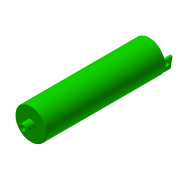
# Autodesk Inventor part: PC3.5-P1
Saved by Autodesk Inventor 2015 (Build 190159000, 159)
## iProperties
Created: 2015-01-13
Part Number: PC3.5-P1
Material: Generic
Document SubType Name: Modeling
Designer: Collin_2
Density: 1 g/cm^3
Appearance: Default
Author: Collin_2
Autodesk Inventor part; units mm, degrees
ref_plane "YZ Plane" through (0, 0, 0) normal (1, 0, 0) x (0, 1, 0)
ref_plane "XZ Plane" through (0, 0, 0) normal (0, 1, 0) x (-1, 0, 0)
ref_plane "XY Plane" through (0, 0, 0) normal (0, 0, 1) x (1, 0, 0)
sketch "Sketch1" plane through (0, 0, 0) normal (0, 1, 0) x (-1, 0, 0)
  line L0 (26.7131, 53.7275) -> (-24.0869, 53.7275)
  line L1 (-24.0869, 53.7275) -> (-24.0869, -136.7725)
  line L2 (-24.0869, -136.7725) -> (26.7131, -136.7725)
  line L3 (26.7131, -136.7725) -> (26.7131, 53.7275)
  line L4 (1.3131, 53.7275) -> (1.3131, -136.7725)
  point P0 (0, 0)
  dimension "d0" = 50.8
  dimension "d1" = 190.5
  constraints: 10 end point, 2 midpoint, 2 parallel, 1 horizontal, 1 perpendicular
  measures "d0" distance of L0.start L0.end
  measures "d1" distance of L2.end L0.start
revolve "Revolution1" add sketch "Sketch1" angle 360 about axis through (-1.3131, 0, 53.7275) along (0, 0, -1) contours L3 L2 L4 L0
sketch "Sketch2" plane through (-1.3131, 0, 53.7275) normal (0, 0, 1) x (1, 0, 0)
  circle A0 centre (0, 0) radius 3.175
  point P0 (1.3131, 0)
  dimension "d3" = 6.35
  constraints: 1 centre point
  measures "d3" diameter of A0
extrude "Extrusion1" cut sketch "Sketch2" against normal blind 88.9
sketch "Sketch3" plane through (-1.3131, 0, -136.7725) normal (0, 0, -1) x (-1, 0, 0)
  circle A0 centre (0, 0) radius 3.175 projected
  circle A1 centre (0, 0) radius 25.4
  circle A2 centre (0, 0) radius 25.4 projected
  line L0 (-24.7072, 5.892) -> (-21.7262, -13.158)
  line L1 (-21.7262, -13.158) -> (-18.5893, -12.6672)
  line L2 (-18.5893, -12.6672) -> (-21.5704, 6.3828)
  line L3 (-21.5704, 6.3828) -> (-24.7072, 5.892)
  line L4 (0.0661, 25.3999) -> (-0.0281, -25.4)
  line L5 (24.7668, 5.8003) -> (21.7152, -13.2386)
  line L6 (21.7152, -13.2386) -> (18.5802, -12.7361)
  line L7 (18.5802, -12.7361) -> (21.6319, 6.3027)
  line L8 (21.6319, 6.3027) -> (24.7668, 5.8003)
  point P0 (-1.3131, 0)
  dimension "d6" = 3.175
  dimension "d7" = 19.05
  constraints: 18 end point, 8 point on circle, 4 symmetric about line, 2 parallel, 1 centre point, 1 coincident, 1 perpendicular
  measures "d6" distance of L1.end L0.end
  measures "d7" vertical distance of L0.start L0.end
extrude "Extrusion2" add sketch "Sketch3" along normal blind 12.7 contours L3 L2 L1 L0 | L8 L5 A1 | A1 L5 L6 L7 L8 | A1 L5 L6
sketch "Sketch4" plane through (20.4131, -13.158, -136.7725) normal (0.9879767, -0.1546027, 0) x (0, 0, -1)
  line L0 (12.7, 19.2818) -> (0, 19.2818)
  line L1 (0, 19.2818) -> (0, 0.2277)
  line L2 (0, 0.2277) -> (12.7, 0.2277)
  line L3 (12.7, 0.2277) -> (12.7, 19.2818)
  circle A0 centre (6.35, 9.5271) radius 3.175
  point P0 (-136.7725, 9.8439)
  dimension "d10" = 6.35
  constraints: 8 end point, 2 parallel, 1 centre point, 1 horizontal, 1 perpendicular
  measures "d10" diameter of A0
extrude "Extrusion3" cut sketch "Sketch4" against normal blind 3149.6 contours A0
sketch "Sketch5" plane through (-1.3131, 0, 53.7275) normal (0, 0, 1) x (1, 0, 0)
  circle A0 centre (0, 0) radius 3.175
  circle A1 centre (0, 0) radius 6.35
  point P0 (1.3131, 0)
  dimension "d13" = 12.7
  constraints: 2 centre point, 1 coincident
  measures "d13" diameter of A1
extrude "Extrusion4" add sketch "Sketch5" along normal blind 12.7
fillet "Fillet1" radius 1.27 4 edges at (-7.6631, 0, 66.4275) (24.0869, 0, 53.7275) (-7.6631, 0, 53.7275) (-4.4881, 0, 66.4275)
body "Solid1"
